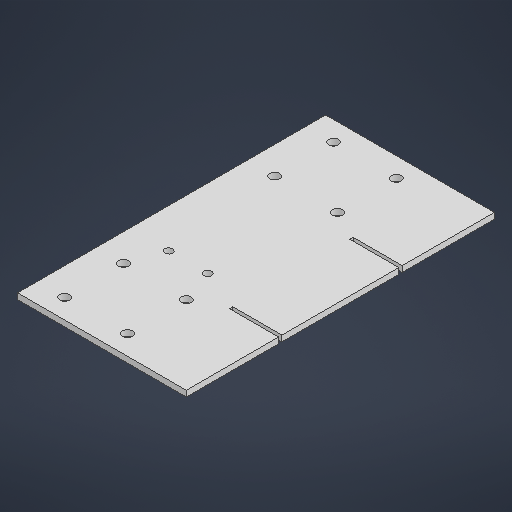
# Autodesk Inventor part: X Axis Base Plate Accurate
Saved by Autodesk Inventor 2025.1 (Build 291241000, 241)
## iProperties
Created: 2025-02-18
Part Number: X Axis Base Plate Accurate
Material: Generic
Document SubType Name: Modeling
Designer: jerem
Density: 1 g/cm^3
Appearance: Default
Author: jerem
## iProperties of the stored document X Axis Base Plate Accurate_3DPrint.ipt
Created: 2025-02-18
Part Number: X Axis Base Plate Accurate_3DPrint
Material: Generic
Document SubType Name: Modeling
Designer: jerem
Density: 1 g/cm^3
Appearance: Default
Author: jerem
Autodesk Inventor part; units mm, degrees
ref_plane "YZ Plane" through (0, 0, 0) normal (1, 0, 0) x (0, 1, 0)
ref_plane "XZ Plane" through (0, 0, 0) normal (0, 1, 0) x (-1, 0, 0)
ref_plane "XY Plane" through (0, 0, 0) normal (0, 0, 1) x (1, 0, 0)
sketch "Sketch1" plane through (0, 0, 0) normal (0, 1, 0) x (-1, 0, 0)
  line L0 (0, 0) -> (-86, 0)
  line L1 (-86, 0) -> (-86, -157)
  line L2 (-86, -157) -> (0, -157)
  line L3 (0, -157) -> (0, 0)
  line L4 (-14, -40) -> (-46, -40) construction
  line L5 (-46, -40) -> (-46, -10) construction
  line L6 (-46, -10) -> (-14, -10) construction
  line L7 (-14, -10) -> (-14, -40) construction
  line L8 (-14, -147) -> (-46, -147) construction
  line L9 (-46, -147) -> (-46, -117) construction
  line L10 (-46, -117) -> (-14, -117) construction
  line L11 (-14, -117) -> (-14, -147) construction
  line L12 (-86, -110) -> (-61, -110)
  line L13 (-61, -110) -> (-61, -108.3)
  line L14 (-61, -108.3) -> (-86, -108.3)
  line L15 (-86, -48.7) -> (-61, -48.7)
  line L16 (-61, -48.7) -> (-61, -47)
  line L17 (-61, -47) -> (-86, -47)
  line L18 (-20, -57) -> (-39.9, -57) construction
  dimension "d0" = 86
  dimension "d1" = 157
  dimension "d2" = 32
  dimension "d3" = 30
  dimension "d4" = 14
  dimension "d5" = 10
  dimension "d6" = 32
  dimension "d7" = 30
  dimension "d8" = 10
  dimension "d9" = 14
  dimension "d10" = 1.7
  dimension "d11" = 1.7
  dimension "d13" = 47
  dimension "d15" = 25
  dimension "d16" = 47
  dimension "d26" = 19.9
  dimension "d27" = 20
  dimension "d28" = 57
  constraints: 38 end point, 6 coincident, 6 horizontal, 6 parallel, 6 perpendicular, 4 point on line, 1 collinear, 1 vertical
  measures "d0" distance of L2.end L1.end
  measures "d1" distance of L1.end L0.end
  measures "d2" distance of L4.start L4.end
  measures "d3" distance of L6.end L4.start
  measures "d4" distance between parallel lines of L3 L7
  measures "d5" distance between parallel lines of L0 L6
  measures "d6" distance of L8.start L8.end
  measures "d7" distance of L10.end L8.start
  measures "d8" distance between parallel lines of L2 L8
  measures "d9" distance between parallel lines of L3 L11
  measures "d10" distance of L12.end L13.end
  measures "d11" distance of L15.end L16.end
  measures "d13" distance between parallel lines of L0 L17
  measures "d15" distance from line of L1 L12.end
  measures "d16" distance between parallel lines of L12 L2
  measures "d26" distance of L18.start L18.end
  measures "d27" distance from line of L3 L18.start
  measures "d28" distance between parallel lines of L0 L18
extrude "Extrusion1" add sketch "Sketch1" along normal blind 3 contours L3 L2 L1 L12 L13 L14 L15 L16 L17 L0
hole "Hole1" at (14, 0, -40) at (46, 0, -40) at (46, 0, -10) at (14, 0, -10) at (14, 0, -147) at (46, 0, -117) at (14, 0, -117) at (46, 0, -147) direction (0, 1, 0) diameter 5 end through all
hole "Hole2" at (20, 0, -57) at (39.9, 0, -57) direction (0, 1, 0) diameter 4 end through all
body "Solid1"
